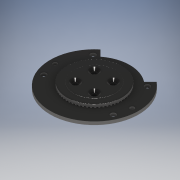
# Autodesk Inventor part: OBROTNICA
Saved by Autodesk Inventor 2017 SP1 (Build 210196100, 196)
## iProperties
Created: 2020-12-24
Part Number: OBROTNICA
Material: Stal nierdzewna, austenityczna
Document SubType Name: Modeling
Designer: Napoleon
Mass: 137.483 g
Surface Area: 122.668 cm^2
Volume: 17.1854 cm^3
Density: 8 g/cm^3
Appearance: Częściowo polerowana
Author: Napoleon
Autodesk Inventor part; units mm, degrees
ref_plane "YZ Plane" through (0, 0, 0) normal (1, 0, 0) x (0, 1, 0)
ref_plane "XZ Plane" through (0, 0, 0) normal (0, 1, 0) x (-1, 0, 0)
ref_plane "XY Plane" through (0, 0, 0) normal (0, 0, 1) x (1, 0, 0)
sketch "Szkic1" plane through (0, 0, 0) normal (0, 0, 1) x (1, 0, 0)
  circle A0 centre (21.5, 20.433648) radius 2
  circle A1 centre (27.5, -12.566352) radius 2
  circle A2 centre (-27.5, -12.566352) radius 2
  circle A3 centre (-21.5, 20.433648) radius 2
  arc A4 (-22.260333, 27.065662) -> (22.201305, 27.068376) centre (-0.027864, 0.033879) ccw
  circle A5 centre (30.5, -0.566352) radius 1.55
  circle A6 centre (-30.5, -0.566352) radius 1.55
  circle A7 centre (30.5, -0.566352) radius 1.625
  circle A8 centre (-0.027864, 0.033879) radius 21.75
  line L0 (-17.289046, 22.094374) -> (-22.260333, 27.065662)
  arc A9 (17.228888, 22.09784) -> (-17.289046, 22.094374) centre (-0.027864, 0.033879) ccw
  line L1 (17.228888, 22.09784) -> (22.201305, 27.068376)
  point P0 (0, 0)
  dimension "d1" = 70
  dimension "d4" = 3.25
  dimension "d5" = 43.5
  constraints: 4 centre point, 4 end point, 4 point on circle, 3 coincident
  measures "d1" diameter of A4
  measures "d4" diameter of A7
  measures "d5" diameter of A8
extrude "Wyciągnięcie proste2" add sketch "Szkic1" along normal blind 2.5 contours L0 A9 L1 A4
sketch "Szkic2" plane through (-0.027864, 0.033879, 2.5) normal (0, 0, 1) x (1, 0.000061, 0)
  circle A0 centre (0, 0) radius 21.75 projected
  circle A1 centre (0, 0) radius 35 projected
  circle A2 centre (0, 0) radius 21.75
  constraints: 1 centre point, 1 coincident
extrude "Wyciągnięcie proste3" add sketch "Szkic2" along normal blind 0.5 separate body contours A0
sketch "Szkic3" plane through (-0.027864, 0.033879, 3) normal (0, 0, 1) x (1, 0, 0)
  circle A0 centre (0, 0) radius 21.75 projected
  circle A1 centre (0, 0) radius 21.9
  dimension "d10" = 43.8
  constraints: 1 centre point, 1 coincident
  measures "d10" diameter of A1
sketch "Szkic3 outline for Wyciągnięcie proste4" plane through (-0.027864, 0.033879, 3) normal (0, 0, 1) x (1, 0, 0)
  circle A0 centre (0, 0) radius 21.75
extrude "Wyciągnięcie proste4" add sketch "Szkic3 outline for Wyciągnięcie proste4" along normal blind 2 and the other way blind 6 separate body
sketch "Szkic4" plane through (-0.027864, 0.033879, 5) normal (0, 0, 1) x (1, 0, 0)
  circle A0 centre (0, 0) radius 21.75 projected
  circle A1 centre (0, 0) radius 16.25
  dimension "d13" = 32.5
  constraints: 1 centre point, 1 coincident
  measures "d13" diameter of A1
extrude "Wyciągnięcie proste5" add sketch "Szkic4" along normal blind 0.15 contours A1 bodies 3
fillet "Zaokrąglenie1" radius 0.1 1 edges at (-16.2779, 0.0339, 5.15)
fillet "Zaokrąglenie2" radius 0.1 1 edges at (-21.7779, 0.0339, 5)
sketch "Szkic5" plane through (-0.027864, 0.033879, 5.15) normal (0, 0, 1) x (1, 0, 0)
  circle A0 centre (7.5, 7.5) radius 3.75
  circle A1 centre (7.5, -7.5) radius 3.75
  circle A2 centre (-7.5, -7.5) radius 3.75
  circle A3 centre (-7.5, 7.5) radius 3.75
  constraints: 4 centre point, 4 coincident
hole "Otwór1" at (7.472136, 7.533879, 5.15) at (7.472136, -7.466121, 5.15) at (-7.527864, -7.466121, 5.15) at (-7.527864, 7.533879, 5.15) direction (0, 0, -1) diameter 4 end through all countersink diameter 7.5 countersink angle 90 bodies 3
thread "Gwint1" size "M4x0.7" class "6H" standard "ANSI Metric M Profile" full length
thread "Gwint2" size "M4x0.7" class "6H" standard "ANSI Metric M Profile" full length
thread "Gwint3" size "M4x0.7" class "6H" standard "ANSI Metric M Profile" full length
thread "Gwint4" size "M4x0.7" class "6H" standard "ANSI Metric M Profile" full length
sketch "Szkic6" plane through (-0.027864, 0.033879, 3) normal (0, 0, 1) x (1, 0, 0)
  point P0 (0.027864, -0.033879)
  point P1 (-7.5, 7.5)
  point P2 (-7.5, -7.5)
  point P3 (7.5, -7.5)
  point P4 (7.5, 7.5)
hole "Otwór2" at (-7.527864, 7.533879, 3) at (-7.527864, -7.466121, 3) at (7.472136, -7.466121, 3) at (7.472136, 7.533879, 3) direction (0, 0, -1) diameter 6 end through all bodies 2
